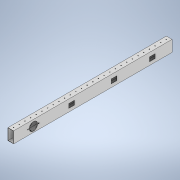
# Autodesk Inventor part: VerseFrame 28in Drive
Saved by Autodesk Inventor 2020 (Build 240168000, 168)
## iProperties
Created: 2020-01-14
Part Number: VerseFrame 28in Drive
Material: Generic
Document SubType Name: Modeling
Designer: aidan
Density: 1 g/cm^3
Appearance: Default
Author: aidan
Autodesk Inventor part; units mm, degrees
ref_plane "YZ Plane" through (0, 0, 0) normal (1, 0, 0) x (0, 1, 0)
ref_plane "XZ Plane" through (0, 0, 0) normal (0, 1, 0) x (-1, 0, 0)
ref_plane "XY Plane" through (0, 0, 0) normal (0, 0, 1) x (1, 0, 0)
sketch "Sketch1" plane through (0, 0, 0) normal (0, 0, 1) x (1, 0, 0)
  line L0 (-12.1708, 16.0073) -> (13.2292, 16.0073)
  line L1 (13.2292, 16.0073) -> (13.2292, -34.7927)
  line L2 (13.2292, -34.7927) -> (-12.1708, -34.7927)
  line L3 (-12.1708, -34.7927) -> (-12.1708, 16.0073)
  line L4 (11.9592, 14.7373) -> (-10.9008, 14.7373)
  line L5 (-10.9008, 14.7373) -> (-10.9008, -33.5227)
  line L6 (-10.9008, -33.5227) -> (11.9592, -33.5227)
  line L7 (11.9592, -33.5227) -> (11.9592, 14.7373)
  point P0 (0, 0)
  dimension "d0" = 25.4
  dimension "d1" = 50.8
  dimension "d2" = 1.27
  constraints: 16 end point, 4 parallel, 2 perpendicular, 1 horizontal, 3 other
  measures "d0" distance of L0.start L0.end
  measures "d1" distance of L0.end L1.end
  measures "d2" distance between parallel lines of L0 L4
extrude "Extrusion1" add sketch "Sketch1" along normal blind 762
sketch "Sketch2" plane through (-12.1708, 16.0073, 0) normal (0, 1, 0) x (1, 0, 0)
  circle A0 centre (12.7, -12.7) radius 1.7272
  line L0 (25.4, 0) -> (0, 0) projected
  line L1 (0, 0) -> (0, -762) projected
  point P0 (12.1708, 0)
  dimension "d5" = 3.4544
  dimension "d6" = 12.7
  dimension "d7" = 12.7
  constraints: 1 centre point
  measures "d5" diameter of A0
  measures "d6" distance from line of L0 A0.centre
  measures "d7" distance from line of L1 A0.centre
extrude "Extrusion2" cut sketch "Sketch2" against normal through all
pattern_linear "Rectangular Pattern1" count 30 spacing 25.4 along (0, 0, 1) of "Extrusion2"
sketch "Sketch3" plane through (-12.1708, 16.0073, 0) normal (0, 1, 0) x (1, 0, 0)
  line L0 (0, 0) -> (25.4, 0)
  line L1 (25.4, 0) -> (25.4, -50.8)
  line L2 (25.4, -50.8) -> (0, -50.8)
  line L3 (0, -50.8) -> (0, 0)
  line L4 (25.4, 0) -> (0, 0) projected
  line L5 (0, 0) -> (0, -762) projected
  point P0 (12.1708, 0)
  dimension "d13" = 25.4
  dimension "d14" = 50.8
  constraints: 8 end point, 2 collinear, 2 parallel, 1 horizontal, 1 perpendicular
  measures "d13" distance of L1.end L2.end
  measures "d14" distance of L0.end L1.end
extrude "Extrusion3" cut sketch "Sketch3" against normal through all
sketch "Sketch4" plane through (13.2292, -34.7927, 762) normal (1, 0, 0) x (0, 0, -1)
  line L0 (-23.8972, 23.8125) -> (751.785, 23.8125) construction
  line L1 (711.2, 50.8) -> (0, 50.8) projected
  line L2 (266.7, 71.9333) -> (266.7, -75.2373) construction
  line L3 (0, 0) -> (0, 50.8) projected
  circle A0 centre (260.35, 23.8125) radius 76.2 construction
  circle A1 centre (450.85, 23.8125) radius 76.2 construction
  line L4 (-23.4814, 26.9875) -> (752.2009, 26.9875) construction
  circle A2 centre (88.9, 23.8125) radius 76.2 construction
  circle A3 centre (622.3, 23.8125) radius 76.2 construction
  line L5 (711.2, 0) -> (711.2, 50.8) projected
  line L6 (438.15, 33.3375) -> (463.55, 33.3375)
  line L7 (463.55, 33.3375) -> (463.55, 14.2875)
  line L8 (463.55, 14.2875) -> (438.15, 14.2875)
  line L9 (438.15, 14.2875) -> (438.15, 33.3375)
  line L10 (438.15, 33.3375) -> (463.55, 14.2875) construction
  line L11 (463.55, 33.3375) -> (438.15, 14.2875) construction
  line L12 (609.6, 33.3375) -> (635, 33.3375)
  line L13 (635, 33.3375) -> (635, 14.2875)
  line L14 (635, 14.2875) -> (609.6, 14.2875)
  line L15 (609.6, 14.2875) -> (609.6, 33.3375)
  line L16 (609.6, 33.3375) -> (635, 14.2875) construction
  line L17 (635, 33.3375) -> (609.6, 14.2875) construction
  line L18 (247.65, 14.2875) -> (273.05, 14.2875)
  line L19 (273.05, 14.2875) -> (273.05, 33.3375)
  line L20 (273.05, 33.3375) -> (247.65, 33.3375)
  line L21 (247.65, 33.3375) -> (247.65, 14.2875)
  line L22 (247.65, 14.2875) -> (273.05, 33.3375) construction
  line L23 (273.05, 14.2875) -> (247.65, 33.3375) construction
  circle A4 centre (88.9, 23.8125) radius 19.05
  circle A5 centre (65.0875, 23.8125) radius 2.4892
  circle A6 centre (112.7125, 23.8125) radius 2.4892
  circle A7 centre (88.9, 23.8125) radius 23.8125 construction
  point P0 (762, 34.7927)
  point P1 (260.35, 23.8125)
  dimension "d18" = 26.9875
  dimension "d25" = 152.4
  dimension "d26" = 3.175
  dimension "d29" = 88.9
  dimension "d34" = 25.4
  dimension "d35" = 19.05
  dimension "d36" = 190.5
  dimension "d37" = 171.45
  dimension "d39" = 47.625
  dimension "d40" = 38.1
  dimension "d41" = 4.9784
  dimension "d42" = 171.45
  constraints: 42 end point, 8 centre point, 7 midpoint, 6 parallel, 6 point on line, 5 horizontal, 4 equal length, 4 equal radius, 3 perpendicular, 2 coincident, 2 point on circle, 1 vertical
  measures "d18" distance between parallel lines of L1 L0
  measures "d25" diameter of A0
  measures "d26" distance between parallel lines of L4 L0
  measures "d29" distance from line of L5 A3.centre
  measures "d34" distance of L12.start L12.end
  measures "d35" distance of L14.end L12.start
  measures "d36" distance of A1.centre A0.centre
  measures "d37" distance of A3.centre A1.centre
  measures "d39" distance of A6.centre A5.centre
  measures "d40" diameter of A4
  measures "d41" diameter of A6
  measures "d42" distance of A0.centre A2.centre
extrude "Extrusion4" cut sketch "Sketch4" against normal blind 25.4
body "Solid1"
